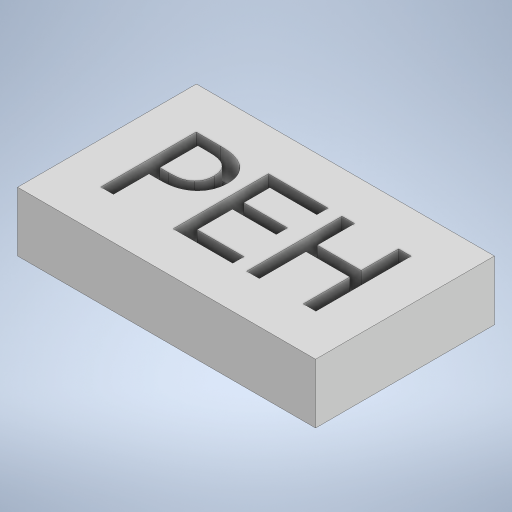
# Autodesk Inventor part: Initial
Saved by Autodesk Inventor 2024 (Build 280153000, 153)
## iProperties
Created: 2024-11-15
Part Number: Initial
Material: 일반
Document SubType Name: Modeling
Designer: SSME0420
Density: 1 g/cm^3
Appearance: 기본값
Author: SSME0420
Autodesk Inventor part; units mm, degrees
ref_plane "YZ Plane" through (0, 0, 0) normal (1, 0, 0) x (0, 1, 0)
ref_plane "XZ Plane" through (0, 0, 0) normal (0, 1, 0) x (-1, 0, 0)
ref_plane "XY Plane" through (0, 0, 0) normal (0, 0, 1) x (1, 0, 0)
sketch "스케치1" plane through (0, 0, 0) normal (0, 1, 0) x (-1, 0, 0)
  line L0 (25, 15) -> (-25, 15)
  line L1 (-25, 15) -> (-25, -15)
  line L2 (-25, -15) -> (25, -15)
  line L3 (25, -15) -> (25, 15)
  line L4 (25, 15) -> (-25, -15) construction
  line L5 (-25, 15) -> (25, -15) construction
  point P0 (0, 0)
  dimension "d0" = 30
  dimension "d1" = 50
  constraints: 12 end point, 2 midpoint, 2 parallel, 1 horizontal, 1 perpendicular
  measures "d0" distance of L0.end L1.end
  measures "d1" distance of L1.end L2.end
extrude "돌출1" add sketch "스케치1" along normal blind 10
sketch "스케치2" plane through (0, 10, 0) normal (0, 1, 0) x (1, 0, 0)
  spline S0 degree 2 poles (-7.9352, 3.1767) (-7.9352, 2.1394) (-8.6742, 0.2723) (-9.3355, -0.376) knots 0 0 0 1 2 2 2
  spline S1 degree 2 poles (-9.3355, -0.376) (-10.1653, -1.1929) (-12.4084, -2.0357) (-14.1199, -2.0357) knots 0 0 0 1 2 2 2
  line L0 (-14.1199, -2.0357) -> (-15.9222, -2.0357)
  line L1 (-15.9222, -2.0357) -> (-15.9222, -8)
  line L2 (-15.9222, -8) -> (-18.0486, -8)
  line L3 (-18.0486, -8) -> (-18.0486, 8)
  line L4 (-18.0486, 8) -> (-14.0292, 8)
  spline S2 degree 2 poles (-14.0292, 8) (-12.6029, 8) (-10.6062, 7.5332) (-9.8412, 7.0016) knots 0 0 0 1 2 2 2
  spline S3 degree 2 poles (-9.8412, 7.0016) (-8.9465, 6.3922) (-7.9352, 4.5122) (-7.9352, 3.1767) knots 0 0 0 1 2 2 2
  spline S4 degree 2 poles (-10.1524, 3.1118) (-10.1524, 3.9417) (-10.7229, 5.1605) (-11.3063, 5.5494) knots 0 0 0 1 2 2 2
  spline S5 degree 2 poles (-11.3063, 5.5494) (-11.812, 5.8865) (-13.1605, 6.1588) (-14.1588, 6.1588) knots 0 0 0 1 2 2 2
  line L5 (-14.1588, 6.1588) -> (-15.9222, 6.1588)
  line L6 (-15.9222, 6.1588) -> (-15.9222, -0.2204)
  line L7 (-15.9222, -0.2204) -> (-14.47, -0.2204)
  spline S6 degree 2 poles (-14.47, -0.2204) (-13.1734, -0.2204) (-11.5786, 0.1945) (-11.06, 0.7391) knots 0 0 0 1 2 2 2
  spline S7 degree 2 poles (-11.06, 0.7391) (-10.5802, 1.2188) (-10.1524, 2.3468) (-10.1524, 3.1118) knots 0 0 0 1 2 2 2
  line L8 (-5.9125, -8) -> (-5.9125, 8)
  line L9 (-5.9125, 8) -> (4.0972, 8)
  line L10 (4.0972, 8) -> (4.0972, 6.107)
  line L11 (4.0972, 6.107) -> (-3.7861, 6.107)
  line L12 (-3.7861, 6.107) -> (-3.7861, 1.7245)
  line L13 (-3.7861, 1.7245) -> (3.5656, 1.7245)
  line L14 (3.5656, 1.7245) -> (3.5656, -0.1686)
  line L15 (3.5656, -0.1686) -> (-3.7861, -0.1686)
  line L16 (-3.7861, -0.1686) -> (-3.7861, -6.107)
  line L17 (-3.7861, -6.107) -> (4.0972, -6.107)
  line L18 (4.0972, -6.107) -> (4.0972, -8)
  line L19 (4.0972, -8) -> (-5.9125, -8)
  line L20 (18.0486, -8) -> (15.9222, -8)
  line L21 (15.9222, -8) -> (15.9222, -0.1686)
  line L22 (15.9222, -0.1686) -> (8.5575, -0.1686)
  line L23 (8.5575, -0.1686) -> (8.5575, -8)
  line L24 (8.5575, -8) -> (6.4311, -8)
  line L25 (6.4311, -8) -> (6.4311, 8)
  line L26 (6.4311, 8) -> (8.5575, 8)
  line L27 (8.5575, 8) -> (8.5575, 1.7245)
  line L28 (8.5575, 1.7245) -> (15.9222, 1.7245)
  line L29 (15.9222, 1.7245) -> (15.9222, 8)
  line L30 (15.9222, 8) -> (18.0486, 8)
  line L31 (18.0486, 8) -> (18.0486, -8)
  point P0 (0, 0)
  point P1 (0, 0)
  constraints: 1 coincident, 1 other
emboss "엠보싱1" sketch "스케치2" operation cut depth 5 direction (0, -1, 0)
